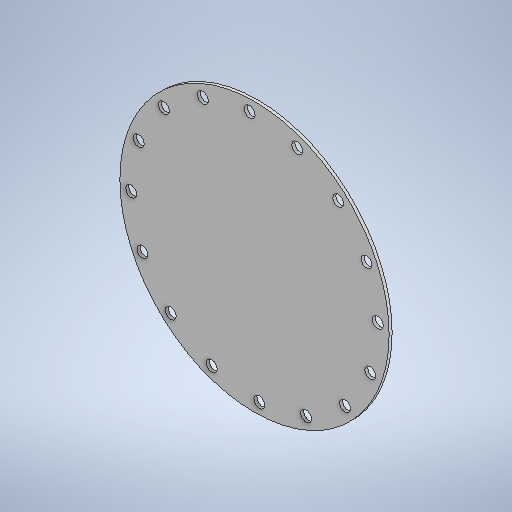
# Autodesk Inventor part: TZS 1212 charging hatch 500 mm
Saved by Autodesk Inventor 2025 (Build 290162010, 162A)
## iProperties
Created: 2025-02-12
Part Number: TZS 1212 charging hatch 500 mm
Material: Steel
Document SubType Name: Sheet Metal
Designer: pokla
Density: 7.85 g/cm^3
Flat Pattern Width: 54 cm
Flat Pattern Length: 54 cm
Flat Pattern Area: 2916 cm^2
Sheet Metal Rule: Default_mm
Sheet Metal Width: 540,000 mm
Sheet Metal Length: 540,000 mm
Sheet Metal Area: 291600,000 mm^2
Appearance: Default
Author: pokla
Autodesk Inventor part; units mm, degrees
ref_plane "YZ Plane" through (0, 0, 0) normal (1, 0, 0) x (0, 1, 0)
ref_plane "XZ Plane" through (0, 0, 0) normal (0, 1, 0) x (-1, 0, 0)
ref_plane "XY Plane" through (0, 0, 0) normal (0, 0, 1) x (1, 0, 0)
sketch "Sketch1" plane through (0, 0, 0) normal (0, 1, 0) x (-1, 0, 0)
  circle A0 centre (0, 0) radius 270
  dimension "d0" = 540
  constraints: 1 centre point, 1 coincident
  measures "d0" diameter of A0
extrude "Extrusion1" add sketch "Sketch1" along normal blind 6
sketch "Sketch2" plane through (0, 6, 0) normal (0, 1, 0) x (1, 0, 0)
  circle A0 centre (0, 0) radius 247.5 construction
  line L0 (0, 0) -> (-247.5, 0)
  line L1 (0, 0) -> (-232.2024, -85.664) construction
  circle A1 centre (-232.2024, -85.664) radius 11
  dimension "d4" = 495
  dimension "d15" = 20.25
  dimension "d16" = 22
  constraints: 4 end point, 2 centre point, 2 coincident, 2 point on circle, 1 horizontal
  measures "d4" diameter of A0
  measures "d15" angle of L1 L0
  measures "d16" diameter of A1
extrude "Cut1" cut sketch "Sketch2" against normal through all
pattern_circular "Circular Pattern1" count 16 over 360 about axis through (0, 0, 0) along (0, 1, 0) of "Cut1"
equation "\"d6\" = Thickness"
equation "\"BendRadius\" = Thickness"
equation "\"BendReliefWidth\" = Thickness"
equation "\"BendReliefDepth\" = 0.5 * Thickness"
equation "\"CornerReliefSize\" = 4 * Thickness"
equation "\"MinimumRemnant\" = 2 * Thickness"
equation "\"TransitionRadius\" = BendRadius"
equation "\"JacobiRadiusSize\" = BendRadius"
equation "\"GapSize\" = Thickness"
equation "\"d5\" = Thickness"
equation "\"Thickness\" = 6"
body "Solid1"
